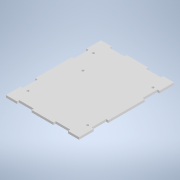
# Autodesk Inventor part: Base
Saved by Autodesk Inventor 2020.3 (Build 243373000, 373)
## iProperties
Created: 2020-08-22
Part Number: Base
Material: Generic
Document SubType Name: Modeling
Designer: Scott Hanson
Density: 1 g/cm^3
Appearance: Default
Width: 100.000 mm
Thickness: 3.000 mm
LengthTabOffset: 20.000 mm
BaseTabWidth: 20.000 mm
WidthTabOffset: 15.000 mm
ScrewDiameter: 3.200 mm
Length: 130.000 mm
Author: Scott Hanson
Autodesk Inventor part; units mm, degrees
ref_plane "YZ Plane" through (0, 0, 0) normal (1, 0, 0) x (0, 1, 0)
ref_plane "XZ Plane" through (0, 0, 0) normal (0, 1, 0) x (-1, 0, 0)
ref_plane "XY Plane" through (0, 0, 0) normal (0, 0, 1) x (1, 0, 0)
sketch "Sketch1" plane through (0, 0, 0) normal (0, 1, 0) x (-1, 0, 0)
  line L0 (0, 0) -> (-100, 0)
  line L1 (-100, 0) -> (-100, -130)
  line L2 (-100, -130) -> (0, -130)
  line L3 (0, -130) -> (0, 0)
  dimension "Length" = 130
  dimension "Width" = 100
  constraints: 8 end point, 2 parallel, 1 horizontal, 1 perpendicular
  measures "Length" distance of L2.end L0.start
  measures "Width" distance of L0.start L0.end
extrude "Baseplate" add sketch "Sketch1" along normal blind 3
sketch "TabsSketch" plane through (0, 3, 0) normal (0, 1, 0) x (1, 0, 0)
  line L0 (0, 130) -> (0, 0) projected
  line L1 (0, 20) -> (3, 20)
  line L2 (3, 20) -> (3, 40)
  line L3 (3, 40) -> (0, 40)
  line L4 (0, 40) -> (0, 20)
  line L5 (0, 90) -> (3, 90)
  line L6 (3, 90) -> (3, 110)
  line L7 (3, 110) -> (0, 110)
  line L8 (0, 110) -> (0, 90)
  line L9 (0, 0) -> (100, 0) projected
  line L10 (100, 130) -> (0, 130) projected
  line L11 (50, 0) -> (50, 130) construction
  line L12 (15, 0) -> (35, 0)
  line L13 (35, 0) -> (35, 3)
  line L14 (35, 3) -> (15, 3)
  line L15 (15, 3) -> (15, 0)
  line L16 (15, 130) -> (35, 130)
  line L17 (35, 130) -> (35, 127)
  line L18 (35, 127) -> (15, 127)
  line L19 (15, 127) -> (15, 130)
  line L20 (100, 130) -> (100, 0)
  line L21 (100, 20) -> (97, 20)
  line L22 (97, 20) -> (97, 40)
  line L23 (97, 40) -> (100, 40)
  line L24 (100, 40) -> (100, 20)
  line L25 (100, 90) -> (97, 90)
  line L26 (97, 90) -> (97, 110)
  line L27 (97, 110) -> (100, 110)
  line L28 (100, 110) -> (100, 90)
  line L29 (100, 0) -> (0, 0)
  line L30 (0, 130) -> (100, 130)
  line L31 (85, 0) -> (65, 0)
  line L32 (65, 0) -> (65, 3)
  line L33 (65, 3) -> (85, 3)
  line L34 (85, 3) -> (85, 0)
  line L35 (85, 130) -> (65, 130)
  line L36 (65, 130) -> (65, 127)
  line L37 (65, 127) -> (85, 127)
  line L38 (85, 127) -> (85, 130)
  point P0 (35, 0)
  point P1 (65, 0)
  point P2 (85, 0)
  point P3 (100, 110)
  point P4 (85, 130)
  point P5 (0, 110)
  point P6 (0, 40)
  dimension "d4" = 3
  dimension "LengthTabOffset" = 20
  dimension "d7" = 20
  dimension "d8" = 20
  dimension "BaseTabWidth" = 20
  dimension "d10" = 50
  dimension "d11" = 3
  dimension "d12" = 3
  dimension "d13" = 20
  dimension "d14" = 20
  dimension "WidthTabOffset" = 15
  dimension "d16" = 30
  constraints: 72 end point, 20 symmetric about line, 12 point on line, 8 parallel, 4 horizontal, 4 perpendicular, 2 midpoint
  measures "d4" distance of L1.start L1.end
  measures "LengthTabOffset" distance from line of L1.end L9
  measures "d7" distance from line of L10 L6.end
  measures "d8" distance of L5.end L6.end
  measures "BaseTabWidth" distance of L1.end L2.end
  measures "d10" distance of L5.end L2.end
  measures "d11" distance of L12.start L14.end
  measures "d12" distance of L18.end L16.start
  measures "d13" distance of L13.end L14.end
  measures "d14" distance of L17.end L18.end
  measures "WidthTabOffset" distance from line of L18.end L0
  measures "d16" distance of L37.start L17.end
extrude "Extrusion2" cut sketch "TabsSketch" against normal through all contours L7 L6 L5 L0 | L10 L17 L18 L19 | L3 L2 L1 L0 | L10 L38 L37 L36 | L15 L14 L13 L9 | L20 L25 L26 L27 | L32 L33 L34 L9 | L20 L21 L22 L23
sketch "Sketch3" plane through (0, 3, 0) normal (0, 1, 0) x (1, 0, 0)
  circle A0 centre (10, 20) radius 1.6
  circle A1 centre (10, 109.5) radius 1.6
  circle A2 centre (91.5, 20) radius 1.6
  circle A3 centre (91.5, 109.5) radius 1.6
  line L0 (0, 20) -> (0, 0) projected
  line L1 (0, 90) -> (0, 40) projected
  line L2 (0, 0) -> (15, 0) projected
  line L3 (35, 0) -> (65, 0) projected
  circle A4 centre (23.5, 81.5) radius 1.6
  dimension "ScrewDiameter" = 3.2
  dimension "d20" = 3.2
  dimension "d21" = 3.2
  dimension "d22" = 3.2
  dimension "d23" = 89.5
  dimension "d24" = 81.5
  dimension "d25" = 89.5
  dimension "d26" = 81.5
  dimension "d27" = 10
  dimension "d28" = 10
  dimension "d29" = 20
  dimension "d30" = 20
  dimension "d31" = 61.5
  dimension "d32" = 68
  dimension "d33" = 3.2
  constraints: 5 centre point
  measures "ScrewDiameter" diameter of A0
  measures "d20" diameter of A1
  measures "d21" diameter of A2
  measures "d22" diameter of A3
  measures "d23" distance of A1.centre A0.centre
  measures "d24" distance of A2.centre A0.centre
  measures "d25" distance of A3.centre A2.centre
  measures "d26" distance of A1.centre A3.centre
  measures "d27" distance from line of A0.centre L0
  measures "d28" distance from line of A1.centre L1
  measures "d29" distance from line of A0.centre L2
  measures "d30" distance from line of A2.centre L3
  measures "d31" vertical distance of A4.centre A2.centre
  measures "d32" horizontal distance of A4.centre A2.centre
  measures "d33" diameter of A4
extrude "PCB Mounting" cut sketch "Sketch3" against normal through all
equation "\"d4\" = Thickness"
equation "\"d7\" = LengthTabOffset"
equation "\"d8\" = BaseTabWidth"
equation "\"d11\" = Thickness"
equation "\"d12\" = Thickness"
equation "\"d13\" = BaseTabWidth"
equation "\"d14\" = BaseTabWidth"
equation "\"d20\" = ScrewDiameter"
equation "\"d21\" = ScrewDiameter"
equation "\"d22\" = d20"
equation "\"d25\" = d23"
equation "\"d26\" = d24"
equation "\"d28\" = d27"
equation "\"d30\" = d29"
equation "\"d33\" = ScrewDiameter"
equation "\"Thickness\" = 3"
body "Solid1"
